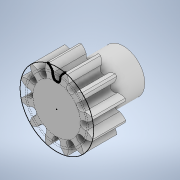
# Autodesk Inventor part: stepper_gear
Saved by Autodesk Inventor 2021 (Build 250183000, 183)
## iProperties
Created: 2021-05-06
Part Number: stepper_gear
Material: Generic
Document SubType Name: Modeling
Designer: froppy
Density: 1 g/cm^3
Appearance: Default
Author: froppy
Autodesk Inventor part; units mm, degrees
ref_plane "YZ Plane" through (0, 0, 0) normal (1, 0, 0) x (0, 1, 0)
ref_plane "XZ Plane" through (0, 0, 0) normal (0, 1, 0) x (-1, 0, 0)
ref_plane "XY Plane" through (0, 0, 0) normal (0, 0, 1) x (1, 0, 0)
sketch "Sketch1" plane through (0, 0, 0) normal (0, 0, 1) x (1, 0, 0)
  spline S0 degree 3 poles (-1.6022, 6.8142) (-1.5555, 6.7733) (-1.4619, 6.6916) (-1.3292, 6.5607) (-1.2029, 6.4236) (-1.0847, 6.2794) (-0.9757, 6.1282) (-0.8941, 5.9959) (-0.8358, 5.8862) (-0.7964, 5.8019) (-0.7611, 5.7155) (-0.744, 5.6558) (-0.7354, 5.6259) knots 0 0 0 0 0.01863 0.037261 0.055891 0.07452 0.093149 0.111776 0.121092 0.130407 0.139721 0.149033 0.149033 0.149033 0.149033
  spline S1 degree 3 poles (-0.7354, 5.6259) (-0.737, 5.5945) (-0.7402, 5.5316) (-0.7403, 5.4371) (-0.7348, 5.3428) (-0.7226, 5.2492) (-0.7067, 5.156) (-0.6818, 5.0648) (-0.6516, 4.9752) (-0.6113, 4.8897) (-0.5633, 4.8082) (-0.5058, 4.7331) (-0.4391, 4.6659) (-0.3756, 4.619) (-0.321, 4.5876) (-0.2638, 4.5613) (-0.1887, 4.5366) (-0.0944, 4.5248) (0, 4.5284) (0.0944, 4.5248) (0.1887, 4.5366) (0.2638, 4.5613) (0.321, 4.5876) (0.3756, 4.619) (0.4391, 4.6659) (0.5058, 4.7331) (0.5633, 4.8082) (0.6113, 4.8897) (0.6516, 4.9752) (0.6818, 5.0648) (0.7067, 5.156) (0.7226, 5.2492) (0.7348, 5.3428) (0.7403, 5.4371) (0.7402, 5.5316) (0.737, 5.5945) (0.7354, 5.6259) knots 0 0 0 0 0.009441 0.018883 0.028326 0.037767 0.047208 0.05665 0.066092 0.075534 0.08497 0.094405 0.10384 0.113275 0.117996 0.122717 0.132151 0.141583 0.151027 0.160471 0.169903 0.179337 0.184058 0.188779 0.198214 0.207648 0.217084 0.22652 0.235962 0.245404 0.254845 0.264287 0.273728 0.283171 0.292613 0.302054 0.302054 0.302054 0.302054
  spline S2 degree 3 poles (0.7354, 5.6259) (0.744, 5.6558) (0.7611, 5.7155) (0.7964, 5.8019) (0.8358, 5.8862) (0.8941, 5.9959) (0.9757, 6.1282) (1.0847, 6.2794) (1.2029, 6.4236) (1.3292, 6.5607) (1.4619, 6.6916) (1.5555, 6.7733) (1.6022, 6.8142) knots 0 0 0 0 0.009312 0.018627 0.027942 0.037257 0.055884 0.074513 0.093143 0.111773 0.130403 0.149033 0.149033 0.149033 0.149033
  circle A0 centre (0, 0) radius 4.5272 construction
  circle A1 centre (0, 0) radius 5.6382 construction
  circle A2 centre (0, 0) radius 6 construction
  circle A3 centre (0, 0) radius 7
  point P0 (-1.4631, 6.6902)
  point P1 (-1.3302, 6.5597)
  point P2 (-1.2043, 6.4224)
  point P3 (-1.0863, 6.2783)
  point P4 (-0.9776, 6.127)
  point P5 (-0.8801, 5.9682)
  point P6 (-0.8365, 5.8859)
  point P7 (-0.797, 5.8015)
  point P8 (-0.7627, 5.715)
  point P9 (-0.7394, 5.5316)
  point P10 (-0.7394, 5.4372)
  point P11 (-0.7337, 5.3429)
  point P12 (-0.722, 5.2492)
  point P13 (-0.7052, 5.1563)
  point P14 (-0.6809, 5.0651)
  point P15 (-0.6499, 4.9759)
  point P16 (-0.61, 4.8903)
  point P17 (-0.5617, 4.8093)
  point P18 (-0.5042, 4.7344)
  point P19 (-0.4375, 4.6677)
  point P20 (-0.3616, 4.6116)
  point P21 (-0.3207, 4.5882)
  point P22 (-0.2778, 4.5684)
  point P23 (-0.188, 4.5396)
  point P24 (-0.0944, 4.5274)
  point P25 (0, 4.5272)
  point P26 (0.0944, 4.5274)
  point P27 (0.188, 4.5396)
  point P28 (0.2778, 4.5684)
  point P29 (0.3207, 4.5882)
  point P30 (0.3616, 4.6116)
  point P31 (0.4375, 4.6677)
  point P32 (0.5042, 4.7344)
  point P33 (0.5617, 4.8093)
  point P34 (0.61, 4.8903)
  point P35 (0.6499, 4.9759)
  point P36 (0.6809, 5.0651)
  point P37 (0.7052, 5.1563)
  point P38 (0.722, 5.2492)
  point P39 (0.7337, 5.3429)
  point P40 (0.7394, 5.4372)
  point P41 (0.7394, 5.5316)
  point P42 (0.7627, 5.715)
  point P43 (0.797, 5.8015)
  point P44 (0.8365, 5.8859)
  point P45 (0.8801, 5.9682)
  point P46 (0.9776, 6.127)
  point P47 (1.0863, 6.2783)
  point P48 (1.2043, 6.4224)
  point P49 (1.3302, 6.5597)
  point P50 (1.4631, 6.6902)
  constraints: 4 centre point, 2 point on circle, 117 other
extrude "Extrusion1" add sketch "Sketch1" against normal blind 6.35
extrude "Extrusion2" cut sketch "Sketch1" against normal through all contours A3 S2 S1 S0 picked at (0.1762, 6.186)
pattern_circular "Circular Pattern1" count 12 over 360 about axis through (0, 0, -10) along (0, 0, 1) of "Extrusion2"
sketch "Sketch2" plane through (0, 0, -6.35) normal (0, 0, -1) x (-1, 0, 0)
  line L0 (1.5, 2) -> (-1.5, 2)
  line L1 (-1.5, 2) -> (-1.5, -2)
  line L2 (-1.5, -2) -> (1.5, -2)
  line L3 (1.5, -2) -> (1.5, 2)
  circle A0 centre (0, 0) radius 2.5
  circle A1 centre (0, 0) radius 4.0875
  point P0 (1.5, -2)
  dimension "d7" = 3
  dimension "d8" = 5
  dimension "d9" = 1.5875
  constraints: 8 end point, 3 point on circle, 2 centre point, 2 coincident, 2 parallel, 1 horizontal, 1 perpendicular
  measures "d7" distance of L1.end L2.end
  measures "d8" diameter of A0
  measures "d9" radial gap between concentric circles of A1 A0
extrude "Extrusion3" add sketch "Sketch2" along normal blind 6.35 contours A0 L3 | L1 A0 | A1
equation "\"d0\" = FaceWidth"
equation "\"Module\" = 1"
equation "\"PressureAngle\" = 20deg"
equation "\"UnitProfileClearance\" = 0.25"
equation "\"UnitRoundRadius\" = 0.35"
equation "\"HeadDiameter\" = 14"
equation "\"RootDiameter\" = 9.05441"
equation "\"BaseDiameter\" = 11.27631"
equation "\"PitchDiameter\" = 12"
equation "\"FaceWidth\" = 6.35"
equation "\"HelixAngle\" = 0"
equation "\"UnitCorrection\" = 0"
equation "\"UnitAddendumModification\" = 0"
equation "\"CircularPitch\" = 3.141593"
equation "\"UnitBacklashShift\" = -0.222794"
equation "\"TotalToolShift\" = -0.22279"
equation "\"IsInternal\" = 0"
body "Solid1"
